Autodesk Fusion 360 part; units mm, degrees
(part 3 of 4)
sketch "草图31" plane through (0, 56.5, 0) normal (0, 1, 0) x (-1, 0, 0)
  line L0 (-115, 90) -> (-115, 0)
  line L1 (-115, 0) -> (125, 0)
  line L2 (125, 0) -> (125, 90)
  line L3 (125, 90) -> (-115, 90)
  line L4 (-106, 14) -> (-110.3301, 11.5)
  line L5 (-110.3301, 11.5) -> (-110.3301, 6.5)
  line L6 (-110.3301, 6.5) -> (-106, 4)
  line L7 (-106, 4) -> (-101.6699, 6.5)
  line L8 (-101.6699, 6.5) -> (-101.6699, 11.5)
  line L9 (-101.6699, 11.5) -> (-106, 14)
  line L10 (-95.3397, 14) -> (-99.6699, 11.5)
  line L11 (-99.6699, 11.5) -> (-99.6699, 6.5)
  line L12 (-99.6699, 6.5) -> (-95.3397, 4)
  line L13 (-95.3397, 4) -> (-91.0096, 6.5)
  line L14 (-91.0096, 6.5) -> (-91.0096, 11.5)
  line L15 (-91.0096, 11.5) -> (-95.3397, 14)
  line L16 (-84.6795, 14) -> (-89.0096, 11.5)
  line L17 (-89.0096, 11.5) -> (-89.0096, 6.5)
  line L18 (-89.0096, 6.5) -> (-84.6795, 4)
  line L19 (-84.6795, 4) -> (-80.3494, 6.5)
  line L20 (-80.3494, 6.5) -> (-80.3494, 11.5)
  line L21 (-80.3494, 11.5) -> (-84.6795, 14)
  line L22 (-74.0192, 14) -> (-78.3494, 11.5)
  line L23 (-78.3494, 11.5) -> (-78.3494, 6.5)
  line L24 (-78.3494, 6.5) -> (-74.0192, 4)
  line L25 (-74.0192, 4) -> (-69.6891, 6.5)
  line L26 (-69.6891, 6.5) -> (-69.6891, 11.5)
  line L27 (-69.6891, 11.5) -> (-74.0192, 14)
  line L28 (-63.359, 14) -> (-67.6891, 11.5)
  line L29 (-67.6891, 11.5) -> (-67.6891, 6.5)
  line L30 (-67.6891, 6.5) -> (-63.359, 4)
  line L31 (-63.359, 4) -> (-59.0289, 6.5)
  line L32 (-59.0289, 6.5) -> (-59.0289, 11.5)
  line L33 (-59.0289, 11.5) -> (-63.359, 14)
  line L34 (-52.6987, 14) -> (-57.0289, 11.5)
  line L35 (-57.0289, 11.5) -> (-57.0289, 6.5)
  line L36 (-57.0289, 6.5) -> (-52.6987, 4)
  line L37 (-52.6987, 4) -> (-48.3686, 6.5)
  line L38 (-48.3686, 6.5) -> (-48.3686, 11.5)
  line L39 (-48.3686, 11.5) -> (-52.6987, 14)
  line L40 (-42.0385, 14) -> (-46.3686, 11.5)
  line L41 (-46.3686, 11.5) -> (-46.3686, 6.5)
  line L42 (-46.3686, 6.5) -> (-42.0385, 4)
  line L43 (-42.0385, 4) -> (-37.7083, 6.5)
  line L44 (-37.7083, 6.5) -> (-37.7083, 11.5)
  line L45 (-37.7083, 11.5) -> (-42.0385, 14)
  line L46 (-31.3782, 14) -> (-35.7083, 11.5)
  line L47 (-35.7083, 11.5) -> (-35.7083, 6.5)
  line L48 (-35.7083, 6.5) -> (-31.3782, 4)
  line L49 (-31.3782, 4) -> (-27.0481, 6.5)
  line L50 (-27.0481, 6.5) -> (-27.0481, 11.5)
  line L51 (-27.0481, 11.5) -> (-31.3782, 14)
  line L52 (-20.718, 14) -> (-25.0481, 11.5)
  line L53 (-25.0481, 11.5) -> (-25.0481, 6.5)
  line L54 (-25.0481, 6.5) -> (-20.718, 4)
  line L55 (-20.718, 4) -> (-16.3878, 6.5)
  line L56 (-16.3878, 6.5) -> (-16.3878, 11.5)
  line L57 (-16.3878, 11.5) -> (-20.718, 14)
  line L58 (-10.0577, 14) -> (-14.3878, 11.5)
  line L59 (-14.3878, 11.5) -> (-14.3878, 6.5)
  line L60 (-14.3878, 6.5) -> (-10.0577, 4)
  line L61 (-10.0577, 4) -> (-5.7276, 6.5)
  line L62 (-5.7276, 6.5) -> (-5.7276, 11.5)
  line L63 (-5.7276, 11.5) -> (-10.0577, 14)
  line L64 (0.6025, 14) -> (-3.7276, 11.5)
  line L65 (-3.7276, 11.5) -> (-3.7276, 6.5)
  line L66 (-3.7276, 6.5) -> (0.6025, 4)
  line L67 (0.6025, 4) -> (4.9327, 6.5)
  line L68 (4.9327, 6.5) -> (4.9327, 11.5)
  line L69 (4.9327, 11.5) -> (0.6025, 14)
  line L70 (11.2628, 14) -> (6.9327, 11.5)
  line L71 (6.9327, 11.5) -> (6.9327, 6.5)
  line L72 (6.9327, 6.5) -> (11.2628, 4)
  line L73 (11.2628, 4) -> (15.5929, 6.5)
  line L74 (15.5929, 6.5) -> (15.5929, 11.5)
  line L75 (15.5929, 11.5) -> (11.2628, 14)
  line L76 (21.923, 14) -> (17.5929, 11.5)
  line L77 (17.5929, 11.5) -> (17.5929, 6.5)
  line L78 (17.5929, 6.5) -> (21.923, 4)
  line L79 (21.923, 4) -> (26.2532, 6.5)
  line L80 (26.2532, 6.5) -> (26.2532, 11.5)
  line L81 (26.2532, 11.5) -> (21.923, 14)
  line L82 (32.5833, 14) -> (28.2532, 11.5)
  line L83 (28.2532, 11.5) -> (28.2532, 6.5)
  line L84 (28.2532, 6.5) -> (32.5833, 4)
  line L85 (32.5833, 4) -> (36.9134, 6.5)
  line L86 (36.9134, 6.5) -> (36.9134, 11.5)
  line L87 (36.9134, 11.5) -> (32.5833, 14)
  line L88 (43.2436, 14) -> (38.9134, 11.5)
  line L89 (38.9134, 11.5) -> (38.9134, 6.5)
  line L90 (38.9134, 6.5) -> (43.2436, 4)
  line L91 (43.2436, 4) -> (47.5737, 6.5)
  line L92 (47.5737, 6.5) -> (47.5737, 11.5)
  line L93 (47.5737, 11.5) -> (43.2436, 14)
  line L94 (53.9038, 14) -> (49.5737, 11.5)
  line L95 (49.5737, 11.5) -> (49.5737, 6.5)
  line L96 (49.5737, 6.5) -> (53.9038, 4)
  line L97 (53.9038, 4) -> (58.2339, 6.5)
  line L98 (58.2339, 6.5) -> (58.2339, 11.5)
  line L99 (58.2339, 11.5) -> (53.9038, 14)
  line L100 (64.5641, 14) -> (60.2339, 11.5)
  line L101 (60.2339, 11.5) -> (60.2339, 6.5)
  line L102 (60.2339, 6.5) -> (64.5641, 4)
  line L103 (64.5641, 4) -> (68.8942, 6.5)
  line L104 (68.8942, 6.5) -> (68.8942, 11.5)
  line L105 (68.8942, 11.5) -> (64.5641, 14)
  line L106 (75.2243, 14) -> (70.8942, 11.5)
  line L107 (70.8942, 11.5) -> (70.8942, 6.5)
  line L108 (70.8942, 6.5) -> (75.2243, 4)
  line L109 (75.2243, 4) -> (79.5544, 6.5)
  line L110 (79.5544, 6.5) -> (79.5544, 11.5)
  line L111 (79.5544, 11.5) -> (75.2243, 14)
  line L112 (85.8846, 14) -> (81.5544, 11.5)
  line L113 (81.5544, 11.5) -> (81.5544, 6.5)
  line L114 (81.5544, 6.5) -> (85.8846, 4)
  line L115 (85.8846, 4) -> (90.2147, 6.5)
  line L116 (90.2147, 6.5) -> (90.2147, 11.5)
  line L117 (90.2147, 11.5) -> (85.8846, 14)
  line L118 (96.5448, 14) -> (92.2147, 11.5)
  line L119 (92.2147, 11.5) -> (92.2147, 6.5)
  line L120 (92.2147, 6.5) -> (96.5448, 4)
  line L121 (96.5448, 4) -> (100.875, 6.5)
  line L122 (100.875, 6.5) -> (100.875, 11.5)
  line L123 (100.875, 11.5) -> (96.5448, 14)
  line L124 (107.2051, 14) -> (102.875, 11.5)
  line L125 (102.875, 11.5) -> (102.875, 6.5)
  line L126 (102.875, 6.5) -> (107.2051, 4)
  line L127 (107.2051, 4) -> (111.5352, 6.5)
  line L128 (111.5352, 6.5) -> (111.5352, 11.5)
  line L129 (111.5352, 11.5) -> (107.2051, 14)
  line L130 (-100.6699, 23.2321) -> (-105, 20.7321)
  line L131 (-105, 20.7321) -> (-105, 15.7321)
  line L132 (-105, 15.7321) -> (-100.6699, 13.2321)
  line L133 (-100.6699, 13.2321) -> (-96.3397, 15.7321)
  line L134 (-96.3397, 15.7321) -> (-96.3397, 20.7321)
  line L135 (-96.3397, 20.7321) -> (-100.6699, 23.2321)
  line L136 (-90.0096, 23.2321) -> (-94.3397, 20.7321)
  line L137 (-94.3397, 20.7321) -> (-94.3397, 15.7321)
  line L138 (-94.3397, 15.7321) -> (-90.0096, 13.2321)
  line L139 (-90.0096, 13.2321) -> (-85.6795, 15.7321)
  line L140 (-85.6795, 15.7321) -> (-85.6795, 20.7321)
  line L141 (-85.6795, 20.7321) -> (-90.0096, 23.2321)
  line L142 (-79.3494, 23.2321) -> (-83.6795, 20.7321)
  line L143 (-83.6795, 20.7321) -> (-83.6795, 15.7321)
  line L144 (-83.6795, 15.7321) -> (-79.3494, 13.2321)
  line L145 (-79.3494, 13.2321) -> (-75.0192, 15.7321)
  line L146 (-75.0192, 15.7321) -> (-75.0192, 20.7321)
  line L147 (-75.0192, 20.7321) -> (-79.3494, 23.2321)
  line L148 (-68.6891, 23.2321) -> (-73.0192, 20.7321)
  line L149 (-73.0192, 20.7321) -> (-73.0192, 15.7321)
  line L150 (-73.0192, 15.7321) -> (-68.6891, 13.2321)
  line L151 (-68.6891, 13.2321) -> (-64.359, 15.7321)
  line L152 (-64.359, 15.7321) -> (-64.359, 20.7321)
  line L153 (-64.359, 20.7321) -> (-68.6891, 23.2321)
  line L154 (-58.0289, 23.2321) -> (-62.359, 20.7321)
  line L155 (-62.359, 20.7321) -> (-62.359, 15.7321)
  line L156 (-62.359, 15.7321) -> (-58.0289, 13.2321)
  line L157 (-58.0289, 13.2321) -> (-53.6987, 15.7321)
  line L158 (-53.6987, 15.7321) -> (-53.6987, 20.7321)
  line L159 (-53.6987, 20.7321) -> (-58.0289, 23.2321)
  line L160 (-47.3686, 23.2321) -> (-51.6987, 20.7321)
  line L161 (-51.6987, 20.7321) -> (-51.6987, 15.7321)
  line L162 (-51.6987, 15.7321) -> (-47.3686, 13.2321)
  line L163 (-47.3686, 13.2321) -> (-43.0385, 15.7321)
  line L164 (-43.0385, 15.7321) -> (-43.0385, 20.7321)
  line L165 (-43.0385, 20.7321) -> (-47.3686, 23.2321)
  line L166 (-36.7083, 23.2321) -> (-41.0385, 20.7321)
  line L167 (-41.0385, 20.7321) -> (-41.0385, 15.7321)
  line L168 (-41.0385, 15.7321) -> (-36.7083, 13.2321)
  line L169 (-36.7083, 13.2321) -> (-32.3782, 15.7321)
  line L170 (-32.3782, 15.7321) -> (-32.3782, 20.7321)
  line L171 (-32.3782, 20.7321) -> (-36.7083, 23.2321)
  line L172 (-26.0481, 23.2321) -> (-30.3782, 20.7321)
  line L173 (-30.3782, 20.7321) -> (-30.3782, 15.7321)
  line L174 (-30.3782, 15.7321) -> (-26.0481, 13.2321)
  line L175 (-26.0481, 13.2321) -> (-21.718, 15.7321)
  line L176 (-21.718, 15.7321) -> (-21.718, 20.7321)
  line L177 (-21.718, 20.7321) -> (-26.0481, 23.2321)
  line L178 (-15.3878, 23.2321) -> (-19.718, 20.7321)
  line L179 (-19.718, 20.7321) -> (-19.718, 15.7321)
  line L180 (-19.718, 15.7321) -> (-15.3878, 13.2321)
  line L181 (-15.3878, 13.2321) -> (-11.0577, 15.7321)
  line L182 (-11.0577, 15.7321) -> (-11.0577, 20.7321)
  line L183 (-11.0577, 20.7321) -> (-15.3878, 23.2321)
  line L184 (-4.7276, 23.2321) -> (-9.0577, 20.7321)
  line L185 (-9.0577, 20.7321) -> (-9.0577, 15.7321)
  line L186 (-9.0577, 15.7321) -> (-4.7276, 13.2321)
  line L187 (-4.7276, 13.2321) -> (-0.3975, 15.7321)
  line L188 (-0.3975, 15.7321) -> (-0.3975, 20.7321)
  line L189 (-0.3975, 20.7321) -> (-4.7276, 23.2321)
  line L190 (5.9327, 23.2321) -> (1.6025, 20.7321)
  line L191 (1.6025, 20.7321) -> (1.6025, 15.7321)
  line L192 (1.6025, 15.7321) -> (5.9327, 13.2321)
  line L193 (5.9327, 13.2321) -> (10.2628, 15.7321)
  line L194 (10.2628, 15.7321) -> (10.2628, 20.7321)
  line L195 (10.2628, 20.7321) -> (5.9327, 23.2321)
  line L196 (16.5929, 23.2321) -> (12.2628, 20.7321)
  line L197 (12.2628, 20.7321) -> (12.2628, 15.7321)
  line L198 (12.2628, 15.7321) -> (16.5929, 13.2321)
  line L199 (16.5929, 13.2321) -> (20.923, 15.7321)
  line L200 (20.923, 15.7321) -> (20.923, 20.7321)
  line L201 (20.923, 20.7321) -> (16.5929, 23.2321)
  line L202 (27.2532, 23.2321) -> (22.923, 20.7321)
  line L203 (22.923, 20.7321) -> (22.923, 15.7321)
  line L204 (22.923, 15.7321) -> (27.2532, 13.2321)
  line L205 (27.2532, 13.2321) -> (31.5833, 15.7321)
  line L206 (31.5833, 15.7321) -> (31.5833, 20.7321)
  line L207 (31.5833, 20.7321) -> (27.2532, 23.2321)
  line L208 (37.9134, 23.2321) -> (33.5833, 20.7321)
  line L209 (33.5833, 20.7321) -> (33.5833, 15.7321)
  line L210 (33.5833, 15.7321) -> (37.9134, 13.2321)
  line L211 (37.9134, 13.2321) -> (42.2436, 15.7321)
  line L212 (42.2436, 15.7321) -> (42.2436, 20.7321)
  line L213 (42.2436, 20.7321) -> (37.9134, 23.2321)
  line L214 (48.5737, 23.2321) -> (44.2436, 20.7321)
  line L215 (44.2436, 20.7321) -> (44.2436, 15.7321)
  line L216 (44.2436, 15.7321) -> (48.5737, 13.2321)
  line L217 (48.5737, 13.2321) -> (52.9038, 15.7321)
  line L218 (52.9038, 15.7321) -> (52.9038, 20.7321)
  line L219 (52.9038, 20.7321) -> (48.5737, 23.2321)
  line L220 (59.2339, 23.2321) -> (54.9038, 20.7321)
  line L221 (54.9038, 20.7321) -> (54.9038, 15.7321)
  line L222 (54.9038, 15.7321) -> (59.2339, 13.2321)
  line L223 (59.2339, 13.2321) -> (63.5641, 15.7321)
  line L224 (63.5641, 15.7321) -> (63.5641, 20.7321)
  line L225 (63.5641, 20.7321) -> (59.2339, 23.2321)
  line L226 (69.8942, 23.2321) -> (65.5641, 20.7321)
  line L227 (65.5641, 20.7321) -> (65.5641, 15.7321)
  line L228 (65.5641, 15.7321) -> (69.8942, 13.2321)
  line L229 (69.8942, 13.2321) -> (74.2243, 15.7321)
  line L230 (74.2243, 15.7321) -> (74.2243, 20.7321)
  line L231 (74.2243, 20.7321) -> (69.8942, 23.2321)
  line L232 (80.5544, 23.2321) -> (76.2243, 20.7321)
  line L233 (76.2243, 20.7321) -> (76.2243, 15.7321)
  line L234 (76.2243, 15.7321) -> (80.5544, 13.2321)
  line L235 (80.5544, 13.2321) -> (84.8846, 15.7321)
  line L236 (84.8846, 15.7321) -> (84.8846, 20.7321)
  line L237 (84.8846, 20.7321) -> (80.5544, 23.2321)
  line L238 (91.2147, 23.2321) -> (86.8846, 20.7321)
  line L239 (86.8846, 20.7321) -> (86.8846, 15.7321)
  line L240 (86.8846, 15.7321) -> (91.2147, 13.2321)
  line L241 (91.2147, 13.2321) -> (95.5448, 15.7321)
  line L242 (95.5448, 15.7321) -> (95.5448, 20.7321)
  line L243 (95.5448, 20.7321) -> (91.2147, 23.2321)
  line L244 (101.875, 23.2321) -> (97.5448, 20.7321)
  line L245 (97.5448, 20.7321) -> (97.5448, 15.7321)
  line L246 (97.5448, 15.7321) -> (101.875, 13.2321)
  line L247 (101.875, 13.2321) -> (106.2051, 15.7321)
  line L248 (106.2051, 15.7321) -> (106.2051, 20.7321)
  line L249 (106.2051, 20.7321) -> (101.875, 23.2321)
  line L250 (112.5352, 23.2321) -> (108.2051, 20.7321)
  line L251 (108.2051, 20.7321) -> (108.2051, 15.7321)
  line L252 (108.2051, 15.7321) -> (112.5352, 13.2321)
  line L253 (112.5352, 13.2321) -> (116.8653, 15.7321)
  line L254 (116.8653, 15.7321) -> (116.8653, 20.7321)
  line L255 (116.8653, 20.7321) -> (112.5352, 23.2321)
  line L256 (-106, 32.4641) -> (-110.3301, 29.9641)
  line L257 (-110.3301, 29.9641) -> (-110.3301, 24.9641)
  line L258 (-110.3301, 24.9641) -> (-106, 22.4641)
  line L259 (-106, 22.4641) -> (-101.6699, 24.9641)
  line L260 (-101.6699, 24.9641) -> (-101.6699, 29.9641)
  line L261 (-101.6699, 29.9641) -> (-106, 32.4641)
  line L262 (-95.3397, 32.4641) -> (-99.6699, 29.9641)
  line L263 (-99.6699, 29.9641) -> (-99.6699, 24.9641)
  line L264 (-99.6699, 24.9641) -> (-95.3397, 22.4641)
  line L265 (-95.3397, 22.4641) -> (-91.0096, 24.9641)
  line L266 (-91.0096, 24.9641) -> (-91.0096, 29.9641)
  line L267 (-91.0096, 29.9641) -> (-95.3397, 32.4641)
  line L268 (-84.6795, 32.4641) -> (-89.0096, 29.9641)
  line L269 (-89.0096, 29.9641) -> (-89.0096, 24.9641)
  line L270 (-89.0096, 24.9641) -> (-84.6795, 22.4641)
  line L271 (-84.6795, 22.4641) -> (-80.3494, 24.9641)
  line L272 (-80.3494, 24.9641) -> (-80.3494, 29.9641)
  line L273 (-80.3494, 29.9641) -> (-84.6795, 32.4641)
  line L274 (-74.0192, 32.4641) -> (-78.3494, 29.9641)
  line L275 (-78.3494, 29.9641) -> (-78.3494, 24.9641)
  line L276 (-78.3494, 24.9641) -> (-74.0192, 22.4641)
  line L277 (-74.0192, 22.4641) -> (-69.6891, 24.9641)
  line L278 (-69.6891, 24.9641) -> (-69.6891, 29.9641)
  line L279 (-69.6891, 29.9641) -> (-74.0192, 32.4641)
  line L280 (-63.359, 32.4641) -> (-67.6891, 29.9641)
  line L281 (-67.6891, 29.9641) -> (-67.6891, 24.9641)
  line L282 (-67.6891, 24.9641) -> (-63.359, 22.4641)
  line L283 (-63.359, 22.4641) -> (-59.0289, 24.9641)
  line L284 (-59.0289, 24.9641) -> (-59.0289, 29.9641)
  line L285 (-59.0289, 29.9641) -> (-63.359, 32.4641)
  line L286 (-52.6987, 32.4641) -> (-57.0289, 29.9641)
  line L287 (-57.0289, 29.9641) -> (-57.0289, 24.9641)
  line L288 (-57.0289, 24.9641) -> (-52.6987, 22.4641)
  line L289 (-52.6987, 22.4641) -> (-48.3686, 24.9641)
  line L290 (-48.3686, 24.9641) -> (-48.3686, 29.9641)
  line L291 (-48.3686, 29.9641) -> (-52.6987, 32.4641)
  line L292 (-42.0385, 32.4641) -> (-46.3686, 29.9641)
  line L293 (-46.3686, 29.9641) -> (-46.3686, 24.9641)
  line L294 (-46.3686, 24.9641) -> (-42.0385, 22.4641)
  line L295 (-42.0385, 22.4641) -> (-37.7083, 24.9641)
  line L296 (-37.7083, 24.9641) -> (-37.7083, 29.9641)
  line L297 (-37.7083, 29.9641) -> (-42.0385, 32.4641)
  line L298 (-31.3782, 32.4641) -> (-35.7083, 29.9641)
  line L299 (-35.7083, 29.9641) -> (-35.7083, 24.9641)
  line L300 (-35.7083, 24.9641) -> (-31.3782, 22.4641)
  line L301 (-31.3782, 22.4641) -> (-27.0481, 24.9641)
  line L302 (-27.0481, 24.9641) -> (-27.0481, 29.9641)
  line L303 (-27.0481, 29.9641) -> (-31.3782, 32.4641)
  line L304 (-20.718, 32.4641) -> (-25.0481, 29.9641)
  line L305 (-25.0481, 29.9641) -> (-25.0481, 24.9641)
  line L306 (-25.0481, 24.9641) -> (-20.718, 22.4641)
  line L307 (-20.718, 22.4641) -> (-16.3878, 24.9641)
  line L308 (-16.3878, 24.9641) -> (-16.3878, 29.9641)
  line L309 (-16.3878, 29.9641) -> (-20.718, 32.4641)
  line L310 (-10.0577, 32.4641) -> (-14.3878, 29.9641)
  line L311 (-14.3878, 29.9641) -> (-14.3878, 24.9641)
  line L312 (-14.3878, 24.9641) -> (-10.0577, 22.4641)
  line L313 (-10.0577, 22.4641) -> (-5.7276, 24.9641)
  line L314 (-5.7276, 24.9641) -> (-5.7276, 29.9641)
  line L315 (-5.7276, 29.9641) -> (-10.0577, 32.4641)
  line L316 (0.6025, 32.4641) -> (-3.7276, 29.9641)
  line L317 (-3.7276, 29.9641) -> (-3.7276, 24.9641)
  line L318 (-3.7276, 24.9641) -> (0.6025, 22.4641)
  line L319 (0.6025, 22.4641) -> (4.9327, 24.9641)
  line L320 (4.9327, 24.9641) -> (4.9327, 29.9641)
  line L321 (4.9327, 29.9641) -> (0.6025, 32.4641)
  line L322 (11.2628, 32.4641) -> (6.9327, 29.9641)
  line L323 (6.9327, 29.9641) -> (6.9327, 24.9641)
  line L324 (6.9327, 24.9641) -> (11.2628, 22.4641)
  line L325 (11.2628, 22.4641) -> (15.5929, 24.9641)
  line L326 (15.5929, 24.9641) -> (15.5929, 29.9641)
  line L327 (15.5929, 29.9641) -> (11.2628, 32.4641)
  line L328 (21.923, 32.4641) -> (17.5929, 29.9641)
  line L329 (17.5929, 29.9641) -> (17.5929, 24.9641)
  line L330 (17.5929, 24.9641) -> (21.923, 22.4641)
  line L331 (21.923, 22.4641) -> (26.2532, 24.9641)
  line L332 (26.2532, 24.9641) -> (26.2532, 29.9641)
  line L333 (26.2532, 29.9641) -> (21.923, 32.4641)
  line L334 (32.5833, 32.4641) -> (28.2532, 29.9641)
  line L335 (28.2532, 29.9641) -> (28.2532, 24.9641)
  line L336 (28.2532, 24.9641) -> (32.5833, 22.4641)
  line L337 (32.5833, 22.4641) -> (36.9134, 24.9641)
  line L338 (36.9134, 24.9641) -> (36.9134, 29.9641)
  line L339 (36.9134, 29.9641) -> (32.5833, 32.4641)
  line L340 (43.2436, 32.4641) -> (38.9134, 29.9641)
  line L341 (38.9134, 29.9641) -> (38.9134, 24.9641)
  line L342 (38.9134, 24.9641) -> (43.2436, 22.4641)
  line L343 (43.2436, 22.4641) -> (47.5737, 24.9641)
  line L344 (47.5737, 24.9641) -> (47.5737, 29.9641)
  line L345 (47.5737, 29.9641) -> (43.2436, 32.4641)
  line L346 (53.9038, 32.4641) -> (49.5737, 29.9641)
  line L347 (49.5737, 29.9641) -> (49.5737, 24.9641)
  line L348 (49.5737, 24.9641) -> (53.9038, 22.4641)
  line L349 (53.9038, 22.4641) -> (58.2339, 24.9641)
  line L350 (58.2339, 24.9641) -> (58.2339, 29.9641)
  line L351 (58.2339, 29.9641) -> (53.9038, 32.4641)
  line L352 (64.5641, 32.4641) -> (60.2339, 29.9641)
  line L353 (60.2339, 29.9641) -> (60.2339, 24.9641)
  line L354 (60.2339, 24.9641) -> (64.5641, 22.4641)
  line L355 (64.5641, 22.4641) -> (68.8942, 24.9641)
  line L356 (68.8942, 24.9641) -> (68.8942, 29.9641)
  line L357 (68.8942, 29.9641) -> (64.5641, 32.4641)
  line L358 (75.2243, 32.4641) -> (70.8942, 29.9641)
  line L359 (70.8942, 29.9641) -> (70.8942, 24.9641)
  line L360 (70.8942, 24.9641) -> (75.2243, 22.4641)
  line L361 (75.2243, 22.4641) -> (79.5544, 24.9641)
  line L362 (79.5544, 24.9641) -> (79.5544, 29.9641)
  line L363 (79.5544, 29.9641) -> (75.2243, 32.4641)
  line L364 (85.8846, 32.4641) -> (81.5544, 29.9641)
  line L365 (81.5544, 29.9641) -> (81.5544, 24.9641)
  line L366 (81.5544, 24.9641) -> (85.8846, 22.4641)
  line L367 (85.8846, 22.4641) -> (90.2147, 24.9641)
  line L368 (90.2147, 24.9641) -> (90.2147, 29.9641)
  line L369 (90.2147, 29.9641) -> (85.8846, 32.4641)
  line L370 (96.5448, 32.4641) -> (92.2147, 29.9641)
  line L371 (92.2147, 29.9641) -> (92.2147, 24.9641)
  line L372 (92.2147, 24.9641) -> (96.5448, 22.4641)
  line L373 (96.5448, 22.4641) -> (100.875, 24.9641)
  line L374 (100.875, 24.9641) -> (100.875, 29.9641)
  line L375 (100.875, 29.9641) -> (96.5448, 32.4641)
  line L376 (107.2051, 32.4641) -> (102.875, 29.9641)
  line L377 (102.875, 29.9641) -> (102.875, 24.9641)
  line L378 (102.875, 24.9641) -> (107.2051, 22.4641)
  line L379 (107.2051, 22.4641) -> (111.5352, 24.9641)
  line L380 (111.5352, 24.9641) -> (111.5352, 29.9641)
  line L381 (111.5352, 29.9641) -> (107.2051, 32.4641)
  line L382 (-100.6699, 41.6962) -> (-105, 39.1962)
  line L383 (-105, 39.1962) -> (-105, 34.1962)
  line L384 (-105, 34.1962) -> (-100.6699, 31.6962)
  line L385 (-100.6699, 31.6962) -> (-96.3397, 34.1962)
  line L386 (-96.3397, 34.1962) -> (-96.3397, 39.1962)
  line L387 (-96.3397, 39.1962) -> (-100.6699, 41.6962)
  line L388 (-90.0096, 41.6962) -> (-94.3397, 39.1962)
  line L389 (-94.3397, 39.1962) -> (-94.3397, 34.1962)
  line L390 (-94.3397, 34.1962) -> (-90.0096, 31.6962)
  line L391 (-90.0096, 31.6962) -> (-85.6795, 34.1962)
  line L392 (-85.6795, 34.1962) -> (-85.6795, 39.1962)
  line L393 (-85.6795, 39.1962) -> (-90.0096, 41.6962)
  line L394 (-79.3494, 41.6962) -> (-83.6795, 39.1962)
  line L395 (-83.6795, 39.1962) -> (-83.6795, 34.1962)
  line L396 (-83.6795, 34.1962) -> (-79.3494, 31.6962)
  line L397 (-79.3494, 31.6962) -> (-75.0192, 34.1962)
  line L398 (-75.0192, 34.1962) -> (-75.0192, 39.1962)
  line L399 (-75.0192, 39.1962) -> (-79.3494, 41.6962)
  line L400 (-68.6891, 41.6962) -> (-73.0192, 39.1962)
  line L401 (-73.0192, 39.1962) -> (-73.0192, 34.1962)
  line L402 (-73.0192, 34.1962) -> (-68.6891, 31.6962)
  line L403 (-68.6891, 31.6962) -> (-64.359, 34.1962)
  line L404 (-64.359, 34.1962) -> (-64.359, 39.1962)
  line L405 (-64.359, 39.1962) -> (-68.6891, 41.6962)
  line L406 (-58.0289, 41.6962) -> (-62.359, 39.1962)
  line L407 (-62.359, 39.1962) -> (-62.359, 34.1962)
  line L408 (-62.359, 34.1962) -> (-58.0289, 31.6962)
  line L409 (-58.0289, 31.6962) -> (-53.6987, 34.1962)
  line L410 (-53.6987, 34.1962) -> (-53.6987, 39.1962)
  line L411 (-53.6987, 39.1962) -> (-58.0289, 41.6962)
  line L412 (-47.3686, 41.6962) -> (-51.6987, 39.1962)
  line L413 (-51.6987, 39.1962) -> (-51.6987, 34.1962)
  line L414 (-51.6987, 34.1962) -> (-47.3686, 31.6962)
  line L415 (-47.3686, 31.6962) -> (-43.0385, 34.1962)
  line L416 (-43.0385, 34.1962) -> (-43.0385, 39.1962)
  line L417 (-43.0385, 39.1962) -> (-47.3686, 41.6962)
  line L418 (-36.7083, 41.6962) -> (-41.0385, 39.1962)
  line L419 (-41.0385, 39.1962) -> (-41.0385, 34.1962)
  line L420 (-41.0385, 34.1962) -> (-36.7083, 31.6962)
  line L421 (-36.7083, 31.6962) -> (-32.3782, 34.1962)
  line L422 (-32.3782, 34.1962) -> (-32.3782, 39.1962)
  line L423 (-32.3782, 39.1962) -> (-36.7083, 41.6962)
  line L424 (-26.0481, 41.6962) -> (-30.3782, 39.1962)
  line L425 (-30.3782, 39.1962) -> (-30.3782, 34.1962)
  line L426 (-30.3782, 34.1962) -> (-26.0481, 31.6962)
  line L427 (-26.0481, 31.6962) -> (-21.718, 34.1962)
  line L428 (-21.718, 34.1962) -> (-21.718, 39.1962)
  line L429 (-21.718, 39.1962) -> (-26.0481, 41.6962)
  line L430 (-15.3878, 41.6962) -> (-19.718, 39.1962)
  line L431 (-19.718, 39.1962) -> (-19.718, 34.1962)
  line L432 (-19.718, 34.1962) -> (-15.3878, 31.6962)
  line L433 (-15.3878, 31.6962) -> (-11.0577, 34.1962)
  line L434 (-11.0577, 34.1962) -> (-11.0577, 39.1962)
  line L435 (-11.0577, 39.1962) -> (-15.3878, 41.6962)
  line L436 (-4.7276, 41.6962) -> (-9.0577, 39.1962)
  line L437 (-9.0577, 39.1962) -> (-9.0577, 34.1962)
  line L438 (-9.0577, 34.1962) -> (-4.7276, 31.6962)
  line L439 (-4.7276, 31.6962) -> (-0.3975, 34.1962)
  line L440 (-0.3975, 34.1962) -> (-0.3975, 39.1962)
  line L441 (-0.3975, 39.1962) -> (-4.7276, 41.6962)
  line L442 (5.9327, 41.6962) -> (1.6025, 39.1962)
  line L443 (1.6025, 39.1962) -> (1.6025, 34.1962)
  line L444 (1.6025, 34.1962) -> (5.9327, 31.6962)
  line L445 (5.9327, 31.6962) -> (10.2628, 34.1962)
  line L446 (10.2628, 34.1962) -> (10.2628, 39.1962)
  line L447 (10.2628, 39.1962) -> (5.9327, 41.6962)
  line L448 (16.5929, 41.6962) -> (12.2628, 39.1962)
  line L449 (12.2628, 39.1962) -> (12.2628, 34.1962)
  line L450 (12.2628, 34.1962) -> (16.5929, 31.6962)
  line L451 (16.5929, 31.6962) -> (20.923, 34.1962)
  line L452 (20.923, 34.1962) -> (20.923, 39.1962)
  line L453 (20.923, 39.1962) -> (16.5929, 41.6962)
  line L454 (27.2532, 41.6962) -> (22.923, 39.1962)
  line L455 (22.923, 39.1962) -> (22.923, 34.1962)
  line L456 (22.923, 34.1962) -> (27.2532, 31.6962)
  line L457 (27.2532, 31.6962) -> (31.5833, 34.1962)
  line L458 (31.5833, 34.1962) -> (31.5833, 39.1962)
  line L459 (31.5833, 39.1962) -> (27.2532, 41.6962)
  line L460 (37.9134, 41.6962) -> (33.5833, 39.1962)
  line L461 (33.5833, 39.1962) -> (33.5833, 34.1962)
  line L462 (33.5833, 34.1962) -> (37.9134, 31.6962)
  line L463 (37.9134, 31.6962) -> (42.2436, 34.1962)
  line L464 (42.2436, 34.1962) -> (42.2436, 39.1962)
  line L465 (42.2436, 39.1962) -> (37.9134, 41.6962)
  line L466 (48.5737, 41.6962) -> (44.2436, 39.1962)
  line L467 (44.2436, 39.1962) -> (44.2436, 34.1962)
  line L468 (44.2436, 34.1962) -> (48.5737, 31.6962)
  line L469 (48.5737, 31.6962) -> (52.9038, 34.1962)
  line L470 (52.9038, 34.1962) -> (52.9038, 39.1962)
  line L471 (52.9038, 39.1962) -> (48.5737, 41.6962)
  line L472 (59.2339, 41.6962) -> (54.9038, 39.1962)
  line L473 (54.9038, 39.1962) -> (54.9038, 34.1962)
  line L474 (54.9038, 34.1962) -> (59.2339, 31.6962)
  line L475 (59.2339, 31.6962) -> (63.5641, 34.1962)
  line L476 (63.5641, 34.1962) -> (63.5641, 39.1962)
  line L477 (63.5641, 39.1962) -> (59.2339, 41.6962)
  line L478 (69.8942, 41.6962) -> (65.5641, 39.1962)
  line L479 (65.5641, 39.1962) -> (65.5641, 34.1962)
  line L480 (65.5641, 34.1962) -> (69.8942, 31.6962)
  line L481 (69.8942, 31.6962) -> (74.2243, 34.1962)
  line L482 (74.2243, 34.1962) -> (74.2243, 39.1962)
  line L483 (74.2243, 39.1962) -> (69.8942, 41.6962)
  line L484 (80.5544, 41.6962) -> (76.2243, 39.1962)
  line L485 (76.2243, 39.1962) -> (76.2243, 34.1962)
  line L486 (76.2243, 34.1962) -> (80.5544, 31.6962)
  line L487 (80.5544, 31.6962) -> (84.8846, 34.1962)
  line L488 (84.8846, 34.1962) -> (84.8846, 39.1962)
  line L489 (84.8846, 39.1962) -> (80.5544, 41.6962)
  line L490 (91.2147, 41.6962) -> (86.8846, 39.1962)
  line L491 (86.8846, 39.1962) -> (86.8846, 34.1962)
  line L492 (86.8846, 34.1962) -> (91.2147, 31.6962)
  line L493 (91.2147, 31.6962) -> (95.5448, 34.1962)
  line L494 (95.5448, 34.1962) -> (95.5448, 39.1962)
  line L495 (95.5448, 39.1962) -> (91.2147, 41.6962)
  line L496 (101.875, 41.6962) -> (97.5448, 39.1962)
  line L497 (97.5448, 39.1962) -> (97.5448, 34.1962)
  line L498 (97.5448, 34.1962) -> (101.875, 31.6962)
  line L499 (101.875, 31.6962) -> (106.2051, 34.1962)
  line L500 (106.2051, 34.1962) -> (106.2051, 39.1962)
  line L501 (106.2051, 39.1962) -> (101.875, 41.6962)
  line L502 (112.5352, 41.6962) -> (108.2051, 39.1962)
  line L503 (108.2051, 39.1962) -> (108.2051, 34.1962)
  line L504 (108.2051, 34.1962) -> (112.5352, 31.6962)
  line L505 (112.5352, 31.6962) -> (116.8653, 34.1962)
  line L506 (116.8653, 34.1962) -> (116.8653, 39.1962)
  line L507 (116.8653, 39.1962) -> (112.5352, 41.6962)
  line L508 (-106, 50.9282) -> (-110.3301, 48.4282)
  line L509 (-110.3301, 48.4282) -> (-110.3301, 43.4282)
  line L510 (-110.3301, 43.4282) -> (-106, 40.9282)
  line L511 (-106, 40.9282) -> (-101.6699, 43.4282)
  line L512 (-101.6699, 43.4282) -> (-101.6699, 48.4282)
  line L513 (-101.6699, 48.4282) -> (-106, 50.9282)
  line L514 (-95.3397, 50.9282) -> (-99.6699, 48.4282)
  line L515 (-99.6699, 48.4282) -> (-99.6699, 43.4282)
  line L516 (-99.6699, 43.4282) -> (-95.3397, 40.9282)
  line L517 (-95.3397, 40.9282) -> (-91.0096, 43.4282)
  line L518 (-91.0096, 43.4282) -> (-91.0096, 48.4282)
  line L519 (-91.0096, 48.4282) -> (-95.3397, 50.9282)
  line L520 (-84.6795, 50.9282) -> (-89.0096, 48.4282)
  line L521 (-89.0096, 48.4282) -> (-89.0096, 43.4282)
  line L522 (-89.0096, 43.4282) -> (-84.6795, 40.9282)
  line L523 (-84.6795, 40.9282) -> (-80.3494, 43.4282)
  line L524 (-80.3494, 43.4282) -> (-80.3494, 48.4282)
  line L525 (-80.3494, 48.4282) -> (-84.6795, 50.9282)
  line L526 (-74.0192, 50.9282) -> (-78.3494, 48.4282)
  line L527 (-78.3494, 48.4282) -> (-78.3494, 43.4282)
  line L528 (-78.3494, 43.4282) -> (-74.0192, 40.9282)
  line L529 (-74.0192, 40.9282) -> (-69.6891, 43.4282)
  line L530 (-69.6891, 43.4282) -> (-69.6891, 48.4282)
  line L531 (-69.6891, 48.4282) -> (-74.0192, 50.9282)
  line L532 (-63.359, 50.9282) -> (-67.6891, 48.4282)
  line L533 (-67.6891, 48.4282) -> (-67.6891, 43.4282)
  line L534 (-67.6891, 43.4282) -> (-63.359, 40.9282)
  line L535 (-63.359, 40.9282) -> (-59.0289, 43.4282)
  line L536 (-59.0289, 43.4282) -> (-59.0289, 48.4282)
  line L537 (-59.0289, 48.4282) -> (-63.359, 50.9282)
  line L538 (-52.6987, 50.9282) -> (-57.0289, 48.4282)
  line L539 (-57.0289, 48.4282) -> (-57.0289, 43.4282)
  line L540 (-57.0289, 43.4282) -> (-52.6987, 40.9282)
  line L541 (-52.6987, 40.9282) -> (-48.3686, 43.4282)
  line L542 (-48.3686, 43.4282) -> (-48.3686, 48.4282)
  line L543 (-48.3686, 48.4282) -> (-52.6987, 50.9282)
  line L544 (-42.0385, 50.9282) -> (-46.3686, 48.4282)
  line L545 (-46.3686, 48.4282) -> (-46.3686, 43.4282)
  line L546 (-46.3686, 43.4282) -> (-42.0385, 40.9282)
  line L547 (-42.0385, 40.9282) -> (-37.7083, 43.4282)
  line L548 (-37.7083, 43.4282) -> (-37.7083, 48.4282)
  line L549 (-37.7083, 48.4282) -> (-42.0385, 50.9282)
  line L550 (-31.3782, 50.9282) -> (-35.7083, 48.4282)
  line L551 (-35.7083, 48.4282) -> (-35.7083, 43.4282)
  line L552 (-35.7083, 43.4282) -> (-31.3782, 40.9282)
  line L553 (-31.3782, 40.9282) -> (-27.0481, 43.4282)
  line L554 (-27.0481, 43.4282) -> (-27.0481, 48.4282)
  line L555 (-27.0481, 48.4282) -> (-31.3782, 50.9282)
  line L556 (-20.718, 50.9282) -> (-25.0481, 48.4282)
  line L557 (-25.0481, 48.4282) -> (-25.0481, 43.4282)
  line L558 (-25.0481, 43.4282) -> (-20.718, 40.9282)
  line L559 (-20.718, 40.9282) -> (-16.3878, 43.4282)
  line L560 (-16.3878, 43.4282) -> (-16.3878, 48.4282)
  line L561 (-16.3878, 48.4282) -> (-20.718, 50.9282)
  line L562 (-10.0577, 50.9282) -> (-14.3878, 48.4282)
  line L563 (-14.3878, 48.4282) -> (-14.3878, 43.4282)
  line L564 (-14.3878, 43.4282) -> (-10.0577, 40.9282)
  line L565 (-10.0577, 40.9282) -> (-5.7276, 43.4282)
  line L566 (-5.7276, 43.4282) -> (-5.7276, 48.4282)
  line L567 (-5.7276, 48.4282) -> (-10.0577, 50.9282)
  line L568 (0.6025, 50.9282) -> (-3.7276, 48.4282)
  line L569 (-3.7276, 48.4282) -> (-3.7276, 43.4282)
  line L570 (-3.7276, 43.4282) -> (0.6025, 40.9282)
  line L571 (0.6025, 40.9282) -> (4.9327, 43.4282)
  line L572 (4.9327, 43.4282) -> (4.9327, 48.4282)
  line L573 (4.9327, 48.4282) -> (0.6025, 50.9282)
  line L574 (11.2628, 50.9282) -> (6.9327, 48.4282)
  line L575 (6.9327, 48.4282) -> (6.9327, 43.4282)
  line L576 (6.9327, 43.4282) -> (11.2628, 40.9282)
  line L577 (11.2628, 40.9282) -> (15.5929, 43.4282)
  line L578 (15.5929, 43.4282) -> (15.5929, 48.4282)
  line L579 (15.5929, 48.4282) -> (11.2628, 50.9282)
  line L580 (21.923, 50.9282) -> (17.5929, 48.4282)
  line L581 (17.5929, 48.4282) -> (17.5929, 43.4282)
  line L582 (17.5929, 43.4282) -> (21.923, 40.9282)
  line L583 (21.923, 40.9282) -> (26.2532, 43.4282)
  line L584 (26.2532, 43.4282) -> (26.2532, 48.4282)
  line L585 (26.2532, 48.4282) -> (21.923, 50.9282)
  line L586 (32.5833, 50.9282) -> (28.2532, 48.4282)
  line L587 (28.2532, 48.4282) -> (28.2532, 43.4282)
  line L588 (28.2532, 43.4282) -> (32.5833, 40.9282)
  line L589 (32.5833, 40.9282) -> (36.9134, 43.4282)
  line L590 (36.9134, 43.4282) -> (36.9134, 48.4282)
  line L591 (36.9134, 48.4282) -> (32.5833, 50.9282)
  line L592 (43.2436, 50.9282) -> (38.9134, 48.4282)
  line L593 (38.9134, 48.4282) -> (38.9134, 43.4282)
  line L594 (38.9134, 43.4282) -> (43.2436, 40.9282)
  line L595 (43.2436, 40.9282) -> (47.5737, 43.4282)
  line L596 (47.5737, 43.4282) -> (47.5737, 48.4282)
  line L597 (47.5737, 48.4282) -> (43.2436, 50.9282)
  line L598 (53.9038, 50.9282) -> (49.5737, 48.4282)
  line L599 (49.5737, 48.4282) -> (49.5737, 43.4282)
  line L600 (49.5737, 43.4282) -> (53.9038, 40.9282)
  line L601 (53.9038, 40.9282) -> (58.2339, 43.4282)
  line L602 (58.2339, 43.4282) -> (58.2339, 48.4282)
  line L603 (58.2339, 48.4282) -> (53.9038, 50.9282)
  line L604 (64.5641, 50.9282) -> (60.2339, 48.4282)
  line L605 (60.2339, 48.4282) -> (60.2339, 43.4282)
  line L606 (60.2339, 43.4282) -> (64.5641, 40.9282)
  line L607 (64.5641, 40.9282) -> (68.8942, 43.4282)
  line L608 (68.8942, 43.4282) -> (68.8942, 48.4282)
  line L609 (68.8942, 48.4282) -> (64.5641, 50.9282)
  line L610 (75.2243, 50.9282) -> (70.8942, 48.4282)
  line L611 (70.8942, 48.4282) -> (70.8942, 43.4282)
  line L612 (70.8942, 43.4282) -> (75.2243, 40.9282)
  line L613 (75.2243, 40.9282) -> (79.5544, 43.4282)
  line L614 (79.5544, 43.4282) -> (79.5544, 48.4282)
  line L615 (79.5544, 48.4282) -> (75.2243, 50.9282)
  line L616 (85.8846, 50.9282) -> (81.5544, 48.4282)
  line L617 (81.5544, 48.4282) -> (81.5544, 43.4282)
  line L618 (81.5544, 43.4282) -> (85.8846, 40.9282)
  line L619 (85.8846, 40.9282) -> (90.2147, 43.4282)
  line L620 (90.2147, 43.4282) -> (90.2147, 48.4282)
  line L621 (90.2147, 48.4282) -> (85.8846, 50.9282)
  line L622 (96.5448, 50.9282) -> (92.2147, 48.4282)
  line L623 (92.2147, 48.4282) -> (92.2147, 43.4282)
  line L624 (92.2147, 43.4282) -> (96.5448, 40.9282)
  line L625 (96.5448, 40.9282) -> (100.875, 43.4282)
  line L626 (100.875, 43.4282) -> (100.875, 48.4282)
  line L627 (100.875, 48.4282) -> (96.5448, 50.9282)
  line L628 (107.2051, 50.9282) -> (102.875, 48.4282)
  line L629 (102.875, 48.4282) -> (102.875, 43.4282)
  line L630 (102.875, 43.4282) -> (107.2051, 40.9282)
  line L631 (107.2051, 40.9282) -> (111.5352, 43.4282)
  line L632 (111.5352, 43.4282) -> (111.5352, 48.4282)
  line L633 (111.5352, 48.4282) -> (107.2051, 50.9282)
  line L634 (-100.6699, 60.1603) -> (-105, 57.6603)
  line L635 (-105, 57.6603) -> (-105, 52.6603)
  line L636 (-105, 52.6603) -> (-100.6699, 50.1603)
  line L637 (-100.6699, 50.1603) -> (-96.3397, 52.6603)
  line L638 (-96.3397, 52.6603) -> (-96.3397, 57.6603)
  line L639 (-96.3397, 57.6603) -> (-100.6699, 60.1603)
  line L640 (-90.0096, 60.1603) -> (-94.3397, 57.6603)
  line L641 (-94.3397, 57.6603) -> (-94.3397, 52.6603)
  line L642 (-94.3397, 52.6603) -> (-90.0096, 50.1603)
  line L643 (-90.0096, 50.1603) -> (-85.6795, 52.6603)
  line L644 (-85.6795, 52.6603) -> (-85.6795, 57.6603)
  line L645 (-85.6795, 57.6603) -> (-90.0096, 60.1603)
  line L646 (-79.3494, 60.1603) -> (-83.6795, 57.6603)
  line L647 (-83.6795, 57.6603) -> (-83.6795, 52.6603)
  line L648 (-83.6795, 52.6603) -> (-79.3494, 50.1603)
  line L649 (-79.3494, 50.1603) -> (-75.0192, 52.6603)
  line L650 (-75.0192, 52.6603) -> (-75.0192, 57.6603)
  line L651 (-75.0192, 57.6603) -> (-79.3494, 60.1603)
  line L652 (-68.6891, 60.1603) -> (-73.0192, 57.6603)
  line L653 (-73.0192, 57.6603) -> (-73.0192, 52.6603)
  line L654 (-73.0192, 52.6603) -> (-68.6891, 50.1603)
  line L655 (-68.6891, 50.1603) -> (-64.359, 52.6603)
  line L656 (-64.359, 52.6603) -> (-64.359, 57.6603)
  line L657 (-64.359, 57.6603) -> (-68.6891, 60.1603)
  line L658 (-58.0289, 60.1603) -> (-62.359, 57.6603)
  line L659 (-62.359, 57.6603) -> (-62.359, 52.6603)
  line L660 (-62.359, 52.6603) -> (-58.0289, 50.1603)
  line L661 (-58.0289, 50.1603) -> (-53.6987, 52.6603)
  line L662 (-53.6987, 52.6603) -> (-53.6987, 57.6603)
  line L663 (-53.6987, 57.6603) -> (-58.0289, 60.1603)
  line L664 (-47.3686, 60.1603) -> (-51.6987, 57.6603)
  line L665 (-51.6987, 57.6603) -> (-51.6987, 52.6603)
  line L666 (-51.6987, 52.6603) -> (-47.3686, 50.1603)
  line L667 (-47.3686, 50.1603) -> (-43.0385, 52.6603)
  line L668 (-43.0385, 52.6603) -> (-43.0385, 57.6603)
  line L669 (-43.0385, 57.6603) -> (-47.3686, 60.1603)
  line L670 (-36.7083, 60.1603) -> (-41.0385, 57.6603)
  line L671 (-41.0385, 57.6603) -> (-41.0385, 52.6603)
  line L672 (-41.0385, 52.6603) -> (-36.7083, 50.1603)
  line L673 (-36.7083, 50.1603) -> (-32.3782, 52.6603)
  line L674 (-32.3782, 52.6603) -> (-32.3782, 57.6603)
  line L675 (-32.3782, 57.6603) -> (-36.7083, 60.1603)
  line L676 (-26.0481, 60.1603) -> (-30.3782, 57.6603)
  line L677 (-30.3782, 57.6603) -> (-30.3782, 52.6603)
  line L678 (-30.3782, 52.6603) -> (-26.0481, 50.1603)
  line L679 (-26.0481, 50.1603) -> (-21.718, 52.6603)
  line L680 (-21.718, 52.6603) -> (-21.718, 57.6603)
  line L681 (-21.718, 57.6603) -> (-26.0481, 60.1603)
  line L682 (-15.3878, 60.1603) -> (-19.718, 57.6603)
  line L683 (-19.718, 57.6603) -> (-19.718, 52.6603)
  line L684 (-19.718, 52.6603) -> (-15.3878, 50.1603)
  line L685 (-15.3878, 50.1603) -> (-11.0577, 52.6603)
  line L686 (-11.0577, 52.6603) -> (-11.0577, 57.6603)
  line L687 (-11.0577, 57.6603) -> (-15.3878, 60.1603)
  line L688 (-4.7276, 60.1603) -> (-9.0577, 57.6603)
  line L689 (-9.0577, 57.6603) -> (-9.0577, 52.6603)
  line L690 (-9.0577, 52.6603) -> (-4.7276, 50.1603)
  line L691 (-4.7276, 50.1603) -> (-0.3975, 52.6603)
  line L692 (-0.3975, 52.6603) -> (-0.3975, 57.6603)
  line L693 (-0.3975, 57.6603) -> (-4.7276, 60.1603)
  line L694 (5.9327, 60.1603) -> (1.6025, 57.6603)
  line L695 (1.6025, 57.6603) -> (1.6025, 52.6603)
  line L696 (1.6025, 52.6603) -> (5.9327, 50.1603)
  line L697 (5.9327, 50.1603) -> (10.2628, 52.6603)
  line L698 (10.2628, 52.6603) -> (10.2628, 57.6603)
  line L699 (10.2628, 57.6603) -> (5.9327, 60.1603)
  line L700 (16.5929, 60.1603) -> (12.2628, 57.6603)
  line L701 (12.2628, 57.6603) -> (12.2628, 52.6603)
  line L702 (12.2628, 52.6603) -> (16.5929, 50.1603)
  line L703 (16.5929, 50.1603) -> (20.923, 52.6603)
  line L704 (20.923, 52.6603) -> (20.923, 57.6603)
  line L705 (20.923, 57.6603) -> (16.5929, 60.1603)
  line L706 (27.2532, 60.1603) -> (22.923, 57.6603)
  line L707 (22.923, 57.6603) -> (22.923, 52.6603)
  line L708 (22.923, 52.6603) -> (27.2532, 50.1603)
  line L709 (27.2532, 50.1603) -> (31.5833, 52.6603)
  line L710 (31.5833, 52.6603) -> (31.5833, 57.6603)
  line L711 (31.5833, 57.6603) -> (27.2532, 60.1603)
  line L712 (37.9134, 60.1603) -> (33.5833, 57.6603)
  line L713 (33.5833, 57.6603) -> (33.5833, 52.6603)
  line L714 (33.5833, 52.6603) -> (37.9134, 50.1603)
  line L715 (37.9134, 50.1603) -> (42.2436, 52.6603)
  line L716 (42.2436, 52.6603) -> (42.2436, 57.6603)
  line L717 (42.2436, 57.6603) -> (37.9134, 60.1603)
  line L718 (48.5737, 60.1603) -> (44.2436, 57.6603)
  line L719 (44.2436, 57.6603) -> (44.2436, 52.6603)
  line L720 (44.2436, 52.6603) -> (48.5737, 50.1603)
  line L721 (48.5737, 50.1603) -> (52.9038, 52.6603)
  line L722 (52.9038, 52.6603) -> (52.9038, 57.6603)
  line L723 (52.9038, 57.6603) -> (48.5737, 60.1603)
  line L724 (59.2339, 60.1603) -> (54.9038, 57.6603)
  line L725 (54.9038, 57.6603) -> (54.9038, 52.6603)
  line L726 (54.9038, 52.6603) -> (59.2339, 50.1603)
  line L727 (59.2339, 50.1603) -> (63.5641, 52.6603)
  line L728 (63.5641, 52.6603) -> (63.5641, 57.6603)
  line L729 (63.5641, 57.6603) -> (59.2339, 60.1603)
  line L730 (69.8942, 60.1603) -> (65.5641, 57.6603)
  line L731 (65.5641, 57.6603) -> (65.5641, 52.6603)
  line L732 (65.5641, 52.6603) -> (69.8942, 50.1603)
  line L733 (69.8942, 50.1603) -> (74.2243, 52.6603)
  line L734 (74.2243, 52.6603) -> (74.2243, 57.6603)
  line L735 (74.2243, 57.6603) -> (69.8942, 60.1603)
  line L736 (80.5544, 60.1603) -> (76.2243, 57.6603)
  line L737 (76.2243, 57.6603) -> (76.2243, 52.6603)
  line L738 (76.2243, 52.6603) -> (80.5544, 50.1603)
  line L739 (80.5544, 50.1603) -> (84.8846, 52.6603)
  line L740 (84.8846, 52.6603) -> (84.8846, 57.6603)
  line L741 (84.8846, 57.6603) -> (80.5544, 60.1603)
  line L742 (91.2147, 60.1603) -> (86.8846, 57.6603)
  line L743 (86.8846, 57.6603) -> (86.8846, 52.6603)
  line L744 (86.8846, 52.6603) -> (91.2147, 50.1603)
  line L745 (91.2147, 50.1603) -> (95.5448, 52.6603)
  line L746 (95.5448, 52.6603) -> (95.5448, 57.6603)
  line L747 (95.5448, 57.6603) -> (91.2147, 60.1603)
  line L748 (101.875, 60.1603) -> (97.5448, 57.6603)
  line L749 (97.5448, 57.6603) -> (97.5448, 52.6603)
  line L750 (97.5448, 52.6603) -> (101.875, 50.1603)
  line L751 (101.875, 50.1603) -> (106.2051, 52.6603)
  line L752 (106.2051, 52.6603) -> (106.2051, 57.6603)
  line L753 (106.2051, 57.6603) -> (101.875, 60.1603)
  line L754 (112.5352, 60.1603) -> (108.2051, 57.6603)
  line L755 (108.2051, 57.6603) -> (108.2051, 52.6603)
  line L756 (108.2051, 52.6603) -> (112.5352, 50.1603)
  line L757 (112.5352, 50.1603) -> (116.8653, 52.6603)
  line L758 (116.8653, 52.6603) -> (116.8653, 57.6603)
  line L759 (116.8653, 57.6603) -> (112.5352, 60.1603)
  line L760 (-106, 69.3923) -> (-110.3301, 66.8923)
  line L761 (-110.3301, 66.8923) -> (-110.3301, 61.8923)
  line L762 (-110.3301, 61.8923) -> (-106, 59.3923)
  line L763 (-106, 59.3923) -> (-101.6699, 61.8923)
  line L764 (-101.6699, 61.8923) -> (-101.6699, 66.8923)
  line L765 (-101.6699, 66.8923) -> (-106, 69.3923)
  line L766 (-95.3397, 69.3923) -> (-99.6699, 66.8923)
  line L767 (-99.6699, 66.8923) -> (-99.6699, 61.8923)
  line L768 (-99.6699, 61.8923) -> (-95.3397, 59.3923)
  line L769 (-95.3397, 59.3923) -> (-91.0096, 61.8923)
  line L770 (-91.0096, 61.8923) -> (-91.0096, 66.8923)
  line L771 (-91.0096, 66.8923) -> (-95.3397, 69.3923)
  line L772 (-84.6795, 69.3923) -> (-89.0096, 66.8923)
  line L773 (-89.0096, 66.8923) -> (-89.0096, 61.8923)
  line L774 (-89.0096, 61.8923) -> (-84.6795, 59.3923)
  line L775 (-84.6795, 59.3923) -> (-80.3494, 61.8923)
  line L776 (-80.3494, 61.8923) -> (-80.3494, 66.8923)
  line L777 (-80.3494, 66.8923) -> (-84.6795, 69.3923)
  line L778 (-74.0192, 69.3923) -> (-78.3494, 66.8923)
  line L779 (-78.3494, 66.8923) -> (-78.3494, 61.8923)
  line L780 (-78.3494, 61.8923) -> (-74.0192, 59.3923)
  line L781 (-74.0192, 59.3923) -> (-69.6891, 61.8923)
  line L782 (-69.6891, 61.8923) -> (-69.6891, 66.8923)
  line L783 (-69.6891, 66.8923) -> (-74.0192, 69.3923)
  line L784 (-63.359, 69.3923) -> (-67.6891, 66.8923)
  line L785 (-67.6891, 66.8923) -> (-67.6891, 61.8923)
  line L786 (-67.6891, 61.8923) -> (-63.359, 59.3923)
  line L787 (-63.359, 59.3923) -> (-59.0289, 61.8923)
  line L788 (-59.0289, 61.8923) -> (-59.0289, 66.8923)
  line L789 (-59.0289, 66.8923) -> (-63.359, 69.3923)
  line L790 (-52.6987, 69.3923) -> (-57.0289, 66.8923)
  line L791 (-57.0289, 66.8923) -> (-57.0289, 61.8923)
  line L792 (-57.0289, 61.8923) -> (-52.6987, 59.3923)
  line L793 (-52.6987, 59.3923) -> (-48.3686, 61.8923)
  line L794 (-48.3686, 61.8923) -> (-48.3686, 66.8923)
  line L795 (-48.3686, 66.8923) -> (-52.6987, 69.3923)
  line L796 (-42.0385, 69.3923) -> (-46.3686, 66.8923)
  line L797 (-46.3686, 66.8923) -> (-46.3686, 61.8923)
  line L798 (-46.3686, 61.8923) -> (-42.0385, 59.3923)
  line L799 (-42.0385, 59.3923) -> (-37.7083, 61.8923)
  line L800 (-37.7083, 61.8923) -> (-37.7083, 66.8923)
  line L801 (-37.7083, 66.8923) -> (-42.0385, 69.3923)
  line L802 (-31.3782, 69.3923) -> (-35.7083, 66.8923)
  line L803 (-35.7083, 66.8923) -> (-35.7083, 61.8923)
  line L804 (-35.7083, 61.8923) -> (-31.3782, 59.3923)
  line L805 (-31.3782, 59.3923) -> (-27.0481, 61.8923)
  line L806 (-27.0481, 61.8923) -> (-27.0481, 66.8923)
  line L807 (-27.0481, 66.8923) -> (-31.3782, 69.3923)
  line L808 (-20.718, 69.3923) -> (-25.0481, 66.8923)
  line L809 (-25.0481, 66.8923) -> (-25.0481, 61.8923)
  line L810 (-25.0481, 61.8923) -> (-20.718, 59.3923)
  line L811 (-20.718, 59.3923) -> (-16.3878, 61.8923)
  line L812 (-16.3878, 61.8923) -> (-16.3878, 66.8923)
  line L813 (-16.3878, 66.8923) -> (-20.718, 69.3923)
  line L814 (-10.0577, 69.3923) -> (-14.3878, 66.8923)
  line L815 (-14.3878, 66.8923) -> (-14.3878, 61.8923)
  line L816 (-14.3878, 61.8923) -> (-10.0577, 59.3923)
  line L817 (-10.0577, 59.3923) -> (-5.7276, 61.8923)
  line L818 (-5.7276, 61.8923) -> (-5.7276, 66.8923)
  line L819 (-5.7276, 66.8923) -> (-10.0577, 69.3923)
  line L820 (0.6025, 69.3923) -> (-3.7276, 66.8923)
  line L821 (-3.7276, 66.8923) -> (-3.7276, 61.8923)
  line L822 (-3.7276, 61.8923) -> (0.6025, 59.3923)
  line L823 (0.6025, 59.3923) -> (4.9327, 61.8923)
  line L824 (4.9327, 61.8923) -> (4.9327, 66.8923)
  line L825 (4.9327, 66.8923) -> (0.6025, 69.3923)
  line L826 (11.2628, 69.3923) -> (6.9327, 66.8923)
  line L827 (6.9327, 66.8923) -> (6.9327, 61.8923)
  line L828 (6.9327, 61.8923) -> (11.2628, 59.3923)
  line L829 (11.2628, 59.3923) -> (15.5929, 61.8923)
  line L830 (15.5929, 61.8923) -> (15.5929, 66.8923)
  line L831 (15.5929, 66.8923) -> (11.2628, 69.3923)
  line L832 (21.923, 69.3923) -> (17.5929, 66.8923)
  line L833 (17.5929, 66.8923) -> (17.5929, 61.8923)
  line L834 (17.5929, 61.8923) -> (21.923, 59.3923)
  line L835 (21.923, 59.3923) -> (26.2532, 61.8923)
  line L836 (26.2532, 61.8923) -> (26.2532, 66.8923)
  line L837 (26.2532, 66.8923) -> (21.923, 69.3923)
  line L838 (32.5833, 69.3923) -> (28.2532, 66.8923)
  line L839 (28.2532, 66.8923) -> (28.2532, 61.8923)
  line L840 (28.2532, 61.8923) -> (32.5833, 59.3923)
  line L841 (32.5833, 59.3923) -> (36.9134, 61.8923)
  line L842 (36.9134, 61.8923) -> (36.9134, 66.8923)
  line L843 (36.9134, 66.8923) -> (32.5833, 69.3923)
  line L844 (43.2436, 69.3923) -> (38.9134, 66.8923)
  line L845 (38.9134, 66.8923) -> (38.9134, 61.8923)
  line L846 (38.9134, 61.8923) -> (43.2436, 59.3923)
  line L847 (43.2436, 59.3923) -> (47.5737, 61.8923)
  line L848 (47.5737, 61.8923) -> (47.5737, 66.8923)
  line L849 (47.5737, 66.8923) -> (43.2436, 69.3923)
  line L850 (53.9038, 69.3923) -> (49.5737, 66.8923)
  line L851 (49.5737, 66.8923) -> (49.5737, 61.8923)
  line L852 (49.5737, 61.8923) -> (53.9038, 59.3923)
  line L853 (53.9038, 59.3923) -> (58.2339, 61.8923)
  line L854 (58.2339, 61.8923) -> (58.2339, 66.8923)
  line L855 (58.2339, 66.8923) -> (53.9038, 69.3923)
  line L856 (64.5641, 69.3923) -> (60.2339, 66.8923)
  line L857 (60.2339, 66.8923) -> (60.2339, 61.8923)
  line L858 (60.2339, 61.8923) -> (64.5641, 59.3923)
  line L859 (64.5641, 59.3923) -> (68.8942, 61.8923)
  line L860 (68.8942, 61.8923) -> (68.8942, 66.8923)
  line L861 (68.8942, 66.8923) -> (64.5641, 69.3923)
  line L862 (75.2243, 69.3923) -> (70.8942, 66.8923)
  line L863 (70.8942, 66.8923) -> (70.8942, 61.8923)
  line L864 (70.8942, 61.8923) -> (75.2243, 59.3923)
  line L865 (75.2243, 59.3923) -> (79.5544, 61.8923)
  line L866 (79.5544, 61.8923) -> (79.5544, 66.8923)
  line L867 (79.5544, 66.8923) -> (75.2243, 69.3923)
  line L868 (85.8846, 69.3923) -> (81.5544, 66.8923)
  line L869 (81.5544, 66.8923) -> (81.5544, 61.8923)
  line L870 (81.5544, 61.8923) -> (85.8846, 59.3923)
  line L871 (85.8846, 59.3923) -> (90.2147, 61.8923)
  line L872 (90.2147, 61.8923) -> (90.2147, 66.8923)
  line L873 (90.2147, 66.8923) -> (85.8846, 69.3923)
  line L874 (96.5448, 69.3923) -> (92.2147, 66.8923)
  line L875 (92.2147, 66.8923) -> (92.2147, 61.8923)
  line L876 (92.2147, 61.8923) -> (96.5448, 59.3923)
  line L877 (96.5448, 59.3923) -> (100.875, 61.8923)
  line L878 (100.875, 61.8923) -> (100.875, 66.8923)
  line L879 (100.875, 66.8923) -> (96.5448, 69.3923)
  line L880 (107.2051, 69.3923) -> (102.875, 66.8923)
  line L881 (102.875, 66.8923) -> (102.875, 61.8923)
  line L882 (102.875, 61.8923) -> (107.2051, 59.3923)
  line L883 (107.2051, 59.3923) -> (111.5352, 61.8923)
  line L884 (111.5352, 61.8923) -> (111.5352, 66.8923)
  line L885 (111.5352, 66.8923) -> (107.2051, 69.3923)
  line L886 (-100.6699, 78.6244) -> (-105, 76.1244)
  line L887 (-105, 76.1244) -> (-105, 71.1244)
  line L888 (-105, 71.1244) -> (-100.6699, 68.6244)
  line L889 (-100.6699, 68.6244) -> (-96.3397, 71.1244)
  line L890 (-96.3397, 71.1244) -> (-96.3397, 76.1244)
  line L891 (-96.3397, 76.1244) -> (-100.6699, 78.6244)
  line L892 (-90.0096, 78.6244) -> (-94.3397, 76.1244)
  line L893 (-94.3397, 76.1244) -> (-94.3397, 71.1244)
  line L894 (-94.3397, 71.1244) -> (-90.0096, 68.6244)
  line L895 (-90.0096, 68.6244) -> (-85.6795, 71.1244)
  line L896 (-85.6795, 71.1244) -> (-85.6795, 76.1244)
  line L897 (-85.6795, 76.1244) -> (-90.0096, 78.6244)
  line L898 (-79.3494, 78.6244) -> (-83.6795, 76.1244)
  line L899 (-83.6795, 76.1244) -> (-83.6795, 71.1244)
  line L900 (-83.6795, 71.1244) -> (-79.3494, 68.6244)
  line L901 (-79.3494, 68.6244) -> (-75.0192, 71.1244)
  line L902 (-75.0192, 71.1244) -> (-75.0192, 76.1244)
  line L903 (-75.0192, 76.1244) -> (-79.3494, 78.6244)
  line L904 (-68.6891, 78.6244) -> (-73.0192, 76.1244)
  line L905 (-73.0192, 76.1244) -> (-73.0192, 71.1244)
  line L906 (-73.0192, 71.1244) -> (-68.6891, 68.6244)
  line L907 (-68.6891, 68.6244) -> (-64.359, 71.1244)
  line L908 (-64.359, 71.1244) -> (-64.359, 76.1244)
  line L909 (-64.359, 76.1244) -> (-68.6891, 78.6244)
  line L910 (-58.0289, 78.6244) -> (-62.359, 76.1244)
  line L911 (-62.359, 76.1244) -> (-62.359, 71.1244)
  line L912 (-62.359, 71.1244) -> (-58.0289, 68.6244)
  line L913 (-58.0289, 68.6244) -> (-53.6987, 71.1244)
  line L914 (-53.6987, 71.1244) -> (-53.6987, 76.1244)
  line L915 (-53.6987, 76.1244) -> (-58.0289, 78.6244)
  line L916 (-47.3686, 78.6244) -> (-51.6987, 76.1244)
  line L917 (-51.6987, 76.1244) -> (-51.6987, 71.1244)
  line L918 (-51.6987, 71.1244) -> (-47.3686, 68.6244)
  line L919 (-47.3686, 68.6244) -> (-43.0385, 71.1244)
  line L920 (-43.0385, 71.1244) -> (-43.0385, 76.1244)
  line L921 (-43.0385, 76.1244) -> (-47.3686, 78.6244)
  line L922 (-36.7083, 78.6244) -> (-41.0385, 76.1244)
  line L923 (-41.0385, 76.1244) -> (-41.0385, 71.1244)
  line L924 (-41.0385, 71.1244) -> (-36.7083, 68.6244)
  line L925 (-36.7083, 68.6244) -> (-32.3782, 71.1244)
  line L926 (-32.3782, 71.1244) -> (-32.3782, 76.1244)
  line L927 (-32.3782, 76.1244) -> (-36.7083, 78.6244)
  line L928 (-26.0481, 78.6244) -> (-30.3782, 76.1244)
  line L929 (-30.3782, 76.1244) -> (-30.3782, 71.1244)
  line L930 (-30.3782, 71.1244) -> (-26.0481, 68.6244)
  line L931 (-26.0481, 68.6244) -> (-21.718, 71.1244)
  line L932 (-21.718, 71.1244) -> (-21.718, 76.1244)
  line L933 (-21.718, 76.1244) -> (-26.0481, 78.6244)
  line L934 (-15.3878, 78.6244) -> (-19.718, 76.1244)
  line L935 (-19.718, 76.1244) -> (-19.718, 71.1244)
  line L936 (-19.718, 71.1244) -> (-15.3878, 68.6244)
  line L937 (-15.3878, 68.6244) -> (-11.0577, 71.1244)
  line L938 (-11.0577, 71.1244) -> (-11.0577, 76.1244)
  line L939 (-11.0577, 76.1244) -> (-15.3878, 78.6244)
  line L940 (-4.7276, 78.6244) -> (-9.0577, 76.1244)
  line L941 (-9.0577, 76.1244) -> (-9.0577, 71.1244)
  line L942 (-9.0577, 71.1244) -> (-4.7276, 68.6244)
  line L943 (-4.7276, 68.6244) -> (-0.3975, 71.1244)
  line L944 (-0.3975, 71.1244) -> (-0.3975, 76.1244)
  line L945 (-0.3975, 76.1244) -> (-4.7276, 78.6244)
  line L946 (5.9327, 78.6244) -> (1.6025, 76.1244)
  line L947 (1.6025, 76.1244) -> (1.6025, 71.1244)
  line L948 (1.6025, 71.1244) -> (5.9327, 68.6244)
  line L949 (5.9327, 68.6244) -> (10.2628, 71.1244)